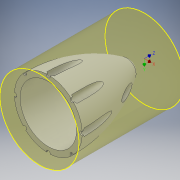
# Autodesk Inventor part: Cabeza
Saved by Autodesk Inventor 2018.3 (Build 223284000, 284)
## iProperties
Created: 2019-03-21
Part Number: Cabeza
Material: Generic
Document SubType Name: Modeling
Designer: Mario
Density: 1 g/cm^3
Appearance: Default
Author: Mario
Autodesk Inventor part; units mm, degrees
ref_plane "YZ Plane" through (0, 0, 0) normal (1, 0, 0) x (0, 1, 0)
sketch "Sketch1" plane through (0, 0, 0) normal (0, 0, 1) x (1, 0, 0)
  line L0 (0, 0) -> (30, 0)
  line L1 (0, 0) -> (0, 73.770422)
  arc A0 (30, 0) -> (8.208955, 69.481206) centre (-91.666667, 0) ccw
  arc A1 (0, 53.770422) -> (8.208955, 69.481206) centre (0, 63.770422) ccw construction
  arc A2 (0, 80) -> (30, 0) centre (-91.666667, 0) ccw construction
  arc A3 (8.208955, 69.481206) -> (0, 80) centre (-91.666667, 0) ccw construction
  arc A4 (8.208955, 69.481206) -> (0, 73.770422) centre (0, 63.770422) ccw
  line L2 (0, 73.770422) -> (0, 80) construction
  line L3 (0, 0) -> (0, 70)
  dimension "d2" = 30
  dimension "d3" = 80
  dimension "d6" = 16.22958
  dimension "d8" = 121.66667
  dimension "d9" = 10
  dimension "d10" = 70
  constraints: 10 point on circle, 8 end point, 5 centre point, 4 point on line, 3 vertical, 1 horizontal, 1 horizontal alignment
  measures "d2" distance of L0.start L0.end
  measures "d3" distance of L0.start L2.end
  measures "d6" distance of A1.centre L2.end
  measures "d8" radius of A0
  measures "d9" radius of A1
  measures "d10" distance of L0.start L3.end
revolve "Revolution1" add sketch "Sketch1" angle 360 about axis through (0, 0, 0) along (0, 1, 0)
shell "Shell1" thickness 5 removed faces 1 at (7.485107, 0, 6.631227)
ref_plane "Work Plane1" through (0, 80, 0) normal (0, -1, 0) x (1, 0, 0)
sketch "Sketch2" plane through (0, 80, 0) normal (0, -1, 0) x (1, 0, 0)
  point P0 (0, 0)
  point P1 (18.257104, 0)
  point P2 (-18.257104, 0)
  dimension "d14" = 18.2571
  dimension "d15" = 18.2571
  constraints: 2 horizontal alignment
  measures "d14" distance of point (18.257, 0) point (0, 0)
  measures "d15" distance of point (0, 0) point (-18.257, 0)
ref_plane "Work Plane2" through (0, 80, 0) normal (0, -1, 0) x (1, 0, 0)
sketch "Sketch5" plane through (0, 80, 0) normal (0, -1, 0) x (1, 0, 0)
  circle A0 centre (0, 0) radius 30
  circle A1 centre (0, 0) radius 29.5 construction
  line L0 (30, 0) -> (-30, 0) construction
  line L1 (0, 30) -> (0, -30) construction
  line L2 (21.213203, -21.213203) -> (-20.85965, 20.85965) construction
  line L3 (21.213203, 21.213203) -> (-21.213203, -21.213203) construction
  point P0 (0, 29.5)
  point P1 (20.85965, 20.85965)
  point P2 (29.5, 0)
  point P3 (20.85965, -20.85965)
  point P4 (0, -29.5)
  point P5 (-20.85965, -20.85965)
  point P6 (-29.5, 0)
  dimension "d33" = 0.5
  dimension "d34" = 45
  dimension "d35" = 45
  constraints: 8 end point, 8 point on line, 6 midpoint, 1 coincident, 1 horizontal, 1 vertical, 18 other
  measures "d34" angle of L3 L0
  measures "d35" angle of L0 L2
hole "Hole2" at (0, 80, 29.5) at (20.85965, 80, 20.85965) at (29.5, 80, 0) at (20.85965, 80, -20.85965) at (0, 80, -29.5) at (-20.85965, 80, -20.85965) at (-29.5, 80, 0) at (-20.85965, 80, 20.85965) direction (0, -1, 0) diameter 6.5 depth 78 tip angle 118
sketch "Sketch6" plane through (0, 80, 0) normal (0, -1, 0) x (1, 0, 0)
  point P0 (0, 0)
  point P1 (20.85965, -20.85965)
  point P2 (29.5, 0)
  point P3 (0, -29.5)
  point P4 (20.85965, 20.85965)
  point P5 (0, 29.5)
  point P6 (-20.85965, 20.85965)
  point P7 (-29.5, 0)
  point P8 (-20.85965, -20.85965)
hole "Hole3" at (20.85965, 80, -20.85965) at (29.5, 80, 0) at (0, 80, -29.5) at (20.85965, 80, 20.85965) at (0, 80, 29.5) at (-20.85965, 80, 20.85965) at (-29.5, 80, 0) at (-20.85965, 80, -20.85965) direction (0, -1, 0) diameter 3.4 end through all clearance for "Socket Head Cap Screw ISO 4762" size "M3" standard "ISO"
hole "Hole4" at (18.257104, 80, 0) at (-18.257104, 80, 0) direction (0, -1, 0) diameter 8 end through all
equation "\"d2\" = R"
equation "\"d3\" = L"
equation "\"d6\" = x0"
equation "\"d8\" = Rho"
equation "\"d9\" = nr"
equation "\"d15\" = d14"
equation "\"R\" = 30"
equation "\"L\" = 80"
equation "\"nr\" = 10"
equation "\"x0\" = 16.229578"
equation "\"Rho\" = 121.666667"
body "Solid1"
